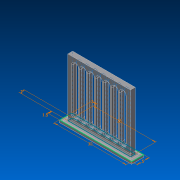
# Autodesk Inventor part: vent test vert
Saved by Autodesk Inventor 2015 (Build 190159000, 159)
## iProperties
Created: 2017-03-16
Part Number: vent test vert
Material: Generic
Document SubType Name: Modeling
Designer: ZigZagJoe
Density: 1 g/cm^3
Appearance: Default
Author: ZigZagJoe
Autodesk Inventor part; units mm, degrees
ref_plane "YZ Plane" through (0, 0, 0) normal (1, 0, 0) x (0, 1, 0)
ref_plane "XZ Plane" through (0, 0, 0) normal (0, 1, 0) x (-1, 0, 0)
ref_plane "XY Plane" through (0, 0, 0) normal (0, 0, 1) x (1, 0, 0)
sketch "Sketch1" plane through (0, 0, 0) normal (0, 0, 1) x (1, 0, 0)
  line L0 (-21.4684, -0.3877) -> (8.5316, -0.3877)
  line L1 (8.5316, -0.3877) -> (8.5316, -5.3877)
  line L2 (8.5316, -5.3877) -> (-21.4684, -5.3877)
  line L3 (-21.4684, -5.3877) -> (-21.4684, -0.3877)
  line L4 (-19.4684, -1.8877) -> (6.5316, -1.8877)
  line L5 (6.5316, -1.8877) -> (6.5316, -3.8877)
  line L6 (6.5316, -3.8877) -> (-19.4684, -3.8877)
  line L7 (-19.4684, -3.8877) -> (-19.4684, -1.8877)
  point P0 (0, 0)
  dimension "d0" = 30
  dimension "d1" = 5
  dimension "d4" = 2
  dimension "d5" = 26
  dimension "d6" = 2
  dimension "d7" = 1.5
  constraints: 16 end point, 4 parallel, 2 horizontal, 2 perpendicular
  measures "d0" distance of L1.end L2.end
  measures "d1" distance of L0.end L1.end
  measures "d4" distance of L6.end L4.start
  measures "d5" distance of L4.start L4.end
  measures "d6" distance between parallel lines of L3 L7
  measures "d7" distance between parallel lines of L2 L6
extrude "Extrusion1" add sketch "Sketch1" along normal blind 24 contours L4 L5 L6 L7
extrude "Extrusion2" add sketch "Sketch1" against normal blind 1 contours L0 L1 L2 L3 | L4 L5 L6 L7
fillet "Fillet1" radius 1 4 edges at (-6.4684, -3.8877, 0) (-19.4684, -2.8877, 0) (-6.4684, -1.8877, 0) (6.5316, -2.8877, 0)
sketch "Sketch2" plane through (-19.4684, -3.8877, 24) normal (0, -1, 0) x (1, 0, 0)
  line L0 (25, -1) -> (1, -1)
  line L1 (1, -1) -> (1, -17)
  line L2 (1, -17) -> (25, -17)
  line L3 (25, -17) -> (25, -1)
  line L4 (0, 0) -> (26, 0) projected
  line L5 (2.3536, -1) -> (7.3536, -1) construction
  line L6 (6.3033, -1) -> (4.182, -3.1213)
  line L7 (4.182, -3.1213) -> (2.0607, -1)
  line L8 (1, -2.0607) -> (3.1213, -4.182)
  line L9 (3.1213, -4.182) -> (1, -6.3033)
  line L10 (1, -6.3033) -> (2.0607, -7.364)
  line L11 (2.0607, -7.364) -> (4.182, -5.2426)
  line L12 (4.182, -5.2426) -> (6.3033, -7.364)
  line L13 (6.3033, -7.364) -> (7.364, -6.3033)
  line L14 (7.364, -6.3033) -> (5.2426, -4.182)
  line L15 (5.2426, -4.182) -> (7.364, -2.0607)
  line L16 (7.364, -2.0607) -> (6.3033, -1)
  line L17 (2.0607, -1) -> (1, -2.0607)
  line L18 (7.364, -2.0607) -> (7.364, -6.3033)
  line L19 (6.3033, -7.364) -> (2.0607, -7.364)
  line L20 (1, -6.3033) -> (1, -2.0607)
  line L21 (2.0607, -1) -> (6.3033, -1)
  line L22 (26, -23) -> (26, 0) projected
  line L23 (0, -23) -> (0, 0) projected
  point P0 (19.4684, -24)
  dimension "d28" = 3
  dimension "d29" = 1.5
  dimension "d30" = 3
  dimension "d31" = 1.5
  dimension "d32" = 3
  dimension "d39" = 6.364
  dimension "d40" = 1
  dimension "d41" = 1
  dimension "d42" = 1
  constraints: 42 end point, 12 point on line, 7 perpendicular, 4 parallel, 2 horizontal, 1 collinear
  measures "d28" distance of L11.end L12.end
  measures "d29" distance of L12.end L13.end
  measures "d30" distance of L14.end L15.end
  measures "d31" distance between parallel lines of L11 L9
  measures "d32" distance of L8.start L8.end
  measures "d39" horizontal distance of L13.end L8.start
  measures "d40" distance between parallel lines of L22 L3
  measures "d41" distance between parallel lines of L23 L20
  measures "d42" distance between parallel lines of L4 L0
extrude "Extrusion3" [suppressed]
pattern_linear "Rectangular Pattern1" [suppressed]
sketch "Sketch3" plane through (-19.4684, -3.8877, 24) normal (0, -1, 0) x (1, 0, 0)
  line L0 (3, -3) -> (3, -21) construction
  line L1 (2, -3) -> (2, -21)
  line L2 (4, -21) -> (4, -3)
  arc A0 (4, -3) -> (2, -3) centre (3, -3) ccw
  arc A1 (2, -21) -> (4, -21) centre (3, -21) ccw
  line L3 (0, 0) -> (26, 0) projected
  line L4 (0, -23) -> (0, 0) projected
  point P0 (19.4684, -24)
  point P1 (3, -12)
  dimension "d43" = 2
  dimension "d44" = 3
  dimension "d45" = 18
  dimension "d48" = 3
  constraints: 8 end point, 4 point on circle, 4 tangent, 2 centre point, 1 midpoint, 1 parallel, 1 vertical
  measures "d43" diameter of A1
  measures "d44" distance from line of L0.start L3
  measures "d45" distance of L0.start L0.end
  measures "d48" distance from line of L4 L0.start
extrude "Extrusion4" cut sketch "Sketch3" against normal blind 2
pattern_linear "Rectangular Pattern2" count 7 spacing 3.3 along (1, 0, 0) of "Extrusion4"
fillet "Fillet2" radius 0.4 56 edges at (-16.4684, -3.8877, 22) (-15.4684, -3.8877, 12) (-16.4684, -3.8877, 2) (-17.4684, -3.8877, 12) (-16.4684, -1.8877, 2) (-15.4684, -1.8877, 12) (-16.4684, -1.8877, 22) (-17.4684, -1.8877, 12) (-14.1684, -3.8877, 12) (-13.1684, -3.8877, 22) (-12.1684, -3.8877, 12) (-13.1684, -3.8877, 2) (-12.1684, -1.8877, 12) (-13.1684, -1.8877, 22) (-14.1684, -1.8877, 12) (-13.1684, -1.8877, 2) (-10.8684, -3.8877, 12) (-9.8684, -3.8877, 22) (-8.8684, -3.8877, 12) (-9.8684, -3.8877, 2) (-8.8684, -1.8877, 12) (-9.8684, -1.8877, 22) (-10.8684, -1.8877, 12) (-9.8684, -1.8877, 2) (-7.5684, -3.8877, 12) (-6.5684, -3.8877, 22) (-5.5684, -3.8877, 12) (-6.5684, -3.8877, 2) (-5.5684, -1.8877, 12) (-6.5684, -1.8877, 22) (-7.5684, -1.8877, 12) (-6.5684, -1.8877, 2) (-4.2684, -3.8877, 12) (-3.2684, -3.8877, 22) (-2.2684, -3.8877, 12) (-3.2684, -3.8877, 2) (-2.2684, -1.8877, 12) (-3.2684, -1.8877, 22) (-4.2684, -1.8877, 12) (-3.2684, -1.8877, 2) (-0.9684, -3.8877, 12) (0.0316, -3.8877, 22) (1.0316, -3.8877, 12) (0.0316, -3.8877, 2) (1.0316, -1.8877, 12) (0.0316, -1.8877, 22) (-0.9684, -1.8877, 12) (0.0316, -1.8877, 2) (2.3316, -3.8877, 12) (3.3316, -3.8877, 22) (4.3316, -3.8877, 12) (3.3316, -3.8877, 2) (4.3316, -1.8877, 12) (3.3316, -1.8877, 22) (2.3316, -1.8877, 12) (3.3316, -1.8877, 2)
equation "\"d28\" = d32"
equation "\"d29\" = d31"
equation "\"d30\" = d32"
body "Solid1"
